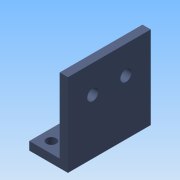
# Autodesk Inventor part: креление кабельканала
Saved by Autodesk Inventor 2017 (Build 210142000, 142)
## iProperties
Part Number: креление кабельканала
Material: Типовые
Document SubType Name: Modeling
Designer: Max
Mass: 2.59249 g
Surface Area: 22.0995 cm^2
Volume: 2.59249 cm^3
Density: 1 g/cm^3
Appearance: Резина — синяя
Author: Max
Autodesk Inventor part; units mm, degrees
ref_plane "YZ Plane" through (0, 0, 0) normal (1, 0, 0) x (0, 1, 0)
ref_plane "XZ Plane" through (0, 0, 0) normal (0, 1, 0) x (-1, 0, 0)
ref_plane "XY Plane" through (0, 0, 0) normal (0, 0, 1) x (1, 0, 0)
sketch "Эскиз1" plane through (0, 0, 0) normal (0, 0, 1) x (1, 0, 0)
  circle A0 centre (142, -81.5) radius 3.75 construction
  circle A1 centre (142, -103.5) radius 3.75 construction
  circle A2 centre (142, -81.5) radius 1.75
  circle A3 centre (142, -103.5) radius 1.75
  line L0 (138, -77.5) -> (152, -77.5)
  line L1 (152, -77.5) -> (152, -107.5)
  line L2 (152, -107.5) -> (138, -107.5)
  line L3 (138, -107.5) -> (138, -77.5)
  line L4 (152, -77.5) -> (149, -77.5)
  line L5 (149, -77.5) -> (149, -107.5)
  line L6 (149, -107.5) -> (152, -107.5)
  line L7 (152, -107.5) -> (152, -77.5)
  point P0 (0, 0)
  dimension "d0" = 3.5
  dimension "d1" = 3.5
  dimension "d2" = 4
  dimension "d3" = 10
  dimension "d4" = 4
  dimension "d5" = 4
  dimension "d6" = 3
  constraints: 16 end point, 4 parallel, 2 centre point, 2 coincident, 2 horizontal, 2 perpendicular, 1 point on line
  measures "d0" diameter of A2
  measures "d1" diameter of A3
  measures "d2" distance from line of L3 A0.centre
  measures "d3" distance from line of A0.centre L1
  measures "d4" distance from line of A0.centre L0
  measures "d5" distance from line of L2 A1.centre
  measures "d6" distance between parallel lines of L1 L5
extrude "Выдавливание1" add sketch "Эскиз1" along normal blind 3
extrude "Выдавливание2" add sketch "Эскиз1" along normal blind 20 contours L0 L1 L2 L5
sketch "Эскиз2" plane through (149, -107.5, 3) normal (-1, 0, 0) x (0, 0, 1)
  circle A0 centre (7, 21) radius 2
  circle A1 centre (7, 9) radius 2
  line L0 (0, 30) -> (17, 30) projected
  line L1 (0, 0) -> (17, 0) projected
  line L2 (17, 30) -> (17, 0) projected
  point P0 (-3, 107.5)
  dimension "d11" = 4
  dimension "d12" = 4
  dimension "d13" = 12
  dimension "d14" = 9
  dimension "d16" = 10
  dimension "d17" = 10
  constraints: 2 centre point
  measures "d11" diameter of A0
  measures "d12" diameter of A1
  measures "d13" distance of A1.centre A0.centre
  measures "d14" distance from line of L0 A0.centre
  measures "d16" distance from line of L2 A0.centre
  measures "d17" distance from line of L2 A1.centre
extrude "Выдавливание3" cut sketch "Эскиз2" against normal blind 10
fillet "Сопряжение1" radius 5 4 edges at (150.5, -77.5, 20) (150.5, -107.5, 20) (138, -77.5, 1.5) (138, -107.5, 1.5)
